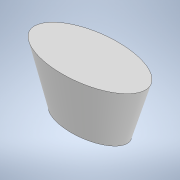
# Autodesk Inventor part: Handle
Saved by Autodesk Inventor 2021 (Build 250183000, 183)
## iProperties
Created: 2021-04-07
Part Number: Handle
Material: Generic
Document SubType Name: Modeling
Designer: Olivi
Density: 1 g/cm^3
Appearance: Default
Author: Olivi
Autodesk Inventor part; units mm, degrees
ref_plane "YZ Plane" through (0, 0, 0) normal (1, 0, 0) x (0, 1, 0)
ref_plane "XZ Plane" through (0, 0, 0) normal (0, 1, 0) x (-1, 0, 0)
ref_plane "XY Plane" through (0, 0, 0) normal (0, 0, 1) x (1, 0, 0)
sketch "Sketch1" plane through (0, 0, 0) normal (0, 0, 1) x (1, 0, 0)
  line L0 (0.8972, 0) -> (0, 0)
  line L1 (0, 0) -> (0, 4.621)
  line L2 (0, 0) -> (0, 20)
  line L3 (0, 20) -> (10, 20)
  line L4 (2.6877, 0) -> (0, 0)
  line L5 (10, 20) -> (6.7227, 0)
  line L6 (6.7227, 0) -> (0, 0)
  dimension "d1" = 20
  dimension "d2" = 10
  constraints: 14 end point, 2 horizontal, 2 vertical, 1 parallel, 1 perpendicular
  measures "d1" distance of L0.end L2.end
  measures "d2" distance of L2.end L3.end
revolve "Revolution1" add sketch "Sketch1" angle 360 about axis through (0, 0, 0) along (0, 1, 0)
scale "Scale1" factors (2, 1, 1) then translate (0, 0, 0) bodies 1
body "Solid1"
